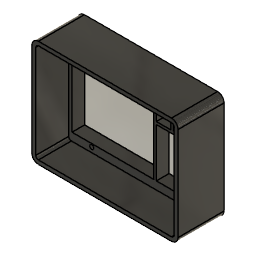
Fibonnaci Body (Autodesk Fusion 360 design; units mm, degrees)
Autodesk Fusion 360 part; units mm, degrees
sketch "Sketch1" plane through (0, 0, 0) normal (0, 1, 0) x (1, 0, 0)
  line L0 (-88.7415, 32.8321) -> (-88.7415, 21.8321)
  line L1 (-88.7415, 21.8321) -> (-77.7415, 21.8321)
  line L2 (-77.7415, 21.8321) -> (-77.7415, 32.8321)
  line L3 (-77.7415, 32.8321) -> (-88.7415, 32.8321)
  line L4 (-77.7415, -30.168) -> (-77.7415, 6.8321)
  line L5 (-77.7415, 19.8321) -> (-88.7415, 19.8321)
  line L6 (-77.7415, 8.8321) -> (-77.7415, 19.8321)
  line L7 (-88.7415, 8.8321) -> (-77.7415, 8.8321)
  line L8 (-88.7415, 19.8321) -> (-88.7415, 8.8321)
  line L9 (-75.7414, 32.8321) -> (-75.7414, -30.168)
  line L10 (-90.7415, 8.8321) -> (-90.7415, 32.8321)
  line L11 (-75.7414, -30.168) -> (-13.7413, -30.168)
  line L12 (-113.7415, 8.8321) -> (-90.7415, 8.8321)
  line L13 (-77.7415, 6.8321) -> (-113.7415, 6.8321)
  line L14 (-90.7415, 32.8321) -> (-113.7415, 32.8321)
  line L15 (-113.7415, -30.168) -> (-77.7415, -30.168)
  line L16 (-13.7413, 32.8321) -> (-75.7414, 32.8321)
  line L17 (-13.7413, 32.8321) -> (-13.7413, -30.168)
  line L18 (-113.7415, 8.8321) -> (-113.7415, 32.8321)
  line L19 (-113.7415, -30.168) -> (-113.7415, 6.8321)
  arc A0 (-27.1914, -32.427) -> (-30.2914, -32.427) centre (-28.7414, -32.427) ccw
  arc A1 (-30.2914, -32.427) -> (-27.1914, -32.427) centre (-28.7414, -32.427) ccw
  arc A2 (-97.1915, -32.427) -> (-100.2915, -32.427) centre (-98.7415, -32.427) ccw
  arc A3 (-100.2915, -32.427) -> (-97.1915, -32.427) centre (-98.7415, -32.427) ccw
  arc A4 (-97.1915, 35.0863) -> (-100.2915, 35.0863) centre (-98.7415, 35.0863) ccw
  arc A5 (-100.2915, 35.0863) -> (-97.1915, 35.0863) centre (-98.7415, 35.0863) ccw
  arc A6 (-30.2914, 35.0863) -> (-27.1914, 35.0863) centre (-28.7414, 35.0863) ccw
  arc A7 (-27.1914, 35.0863) -> (-30.2914, 35.0863) centre (-28.7414, 35.0863) ccw
  line L20 (-118.7415, 6.8321) -> (-118.7415, 8.8321)
  line L21 (-12.7414, 33.8297) -> (-114.7414, 33.8297)
  line L22 (-114.7414, 33.8297) -> (-114.7414, -31.1703)
  line L23 (-114.7414, -31.1703) -> (-12.7414, -31.1703)
  line L24 (-12.7414, -31.1703) -> (-12.7414, 33.8297)
  line L25 (-114.2414, -39.1703) -> (-13.2414, -39.1703)
  line L26 (-8.2414, -34.1703) -> (-8.2414, 36.8297)
  line L27 (-13.2414, 41.8297) -> (-114.2414, 41.8297)
  line L28 (-119.2414, 36.8297) -> (-119.2414, -34.1703)
  arc A8 (-114.2414, 41.8297) -> (-119.2414, 36.8297) centre (-114.2414, 36.8297) ccw
  arc A9 (-8.2414, 36.8297) -> (-13.2414, 41.8297) centre (-13.2414, 36.8297) ccw
  arc A10 (-119.2414, -34.1703) -> (-114.2414, -39.1703) centre (-114.2414, -34.1703) ccw
  arc A11 (-13.2414, -39.1703) -> (-8.2414, -34.1703) centre (-13.2414, -34.1703) ccw
  point P0 (-63.7414, 1.3297)
  dimension "d10" = 102
  dimension "d11" = 65
  dimension "d15" = 5
  constraint horizontal L21
  constraint perpendicular L21 L22
  constraint parallel L21 L23
  constraint parallel L22 L24
  constraint tangent L28 A8
  constraint tangent L27 A8
  constraint tangent L27 A9
  constraint tangent L26 A9
  constraint equal A8 A9
  constraint tangent L28 A10
  constraint tangent L25 A10
  constraint equal A8 A10
  constraint tangent L26 A11
  constraint tangent L25 A11
  constraint equal A8 A11
  measures "d10" distance of L22.end L23.end
  measures "d11" distance of L21.end L22.end
  measures "d15" radius of A8
extrude "Extrude4" add sketch "Sketch1" against normal blind 10 contours A0 A2 A5 A6 L21 L22 L23 L24 | L25 L26 L27 L28 A8 A9 A10 A11 makes body 1
extrude "Extrude5" add sketch "Sketch1" against normal blind 0.4 separate body contours L9 L11 L16 L17 makes body 2
extrude "Extrude6" add sketch "Sketch1" against normal blind 0.4 separate body contours L0 L1 L2 L3 makes body 3
extrude "Extrude7" add sketch "Sketch1" against normal blind 0.4 separate body contours L10 L12 L14 L18 makes body 4
extrude "Extrude8" add sketch "Sketch1" against normal blind 0.4 separate body contours L5 L6 L7 L8 makes body 5
extrude "Extrude9" add sketch "Sketch1" against normal blind 0.4 separate body contours L4 L13 L15 L19 makes body 6
extrude "Extrude10" add sketch "Sketch1" against normal blind 15 contours A0 A1 L23 | A0 L23 | A2 L23 | A2 A3 L23 | A6 A7 L21 | A6 L21 | A4 A5 L21 | A5 L21 bodies 1
sketch "Sketch6" plane through (0, -10, 0) normal (0, -1, 0) x (1, 0, 0)
  line L0 (-90.7415, -8.8321) -> (-90.7415, -32.8321)
  line L1 (-90.7415, -32.8321) -> (-113.7415, -32.8321)
  line L2 (-113.7415, -32.8321) -> (-113.7415, -8.8321)
  line L3 (-113.7415, -8.8321) -> (-90.7415, -8.8321)
  line L4 (-77.7415, 30.168) -> (-77.7415, -6.8321)
  line L5 (-77.7415, -6.8321) -> (-113.7415, -6.8321)
  line L6 (-113.7415, -6.8321) -> (-113.7415, 30.168)
  line L7 (-113.7415, 30.168) -> (-77.7415, 30.168)
  line L8 (-88.7415, -19.8321) -> (-88.7415, -8.8321)
  line L9 (-88.7415, -8.8321) -> (-77.7415, -8.8321)
  line L10 (-77.7415, -8.8321) -> (-77.7415, -19.8321)
  line L11 (-77.7415, -19.8321) -> (-88.7415, -19.8321)
  line L12 (-77.7415, -32.8321) -> (-88.7415, -32.8321)
  line L13 (-88.7415, -32.8321) -> (-88.7415, -21.8321)
  line L14 (-88.7415, -21.8321) -> (-77.7415, -21.8321)
  line L15 (-77.7415, -21.8321) -> (-77.7415, -32.8321)
  line L16 (-75.7414, -32.8321) -> (-75.7414, 30.168)
  line L17 (-75.7414, 30.168) -> (-13.7413, 30.168)
  line L18 (-13.7413, 30.168) -> (-13.7413, -32.8321)
  line L19 (-13.7413, -32.8321) -> (-75.7414, -32.8321)
  arc A0 (-8.2414, 34.1703) -> (-13.2414, 39.1703) centre (-13.2414, 34.1703) ccw
  line L20 (-13.2414, 39.1703) -> (-114.2414, 39.1703)
  arc A1 (-114.2414, 39.1703) -> (-119.2414, 34.1703) centre (-114.2414, 34.1703) ccw
  line L21 (-119.2414, 34.1703) -> (-119.2414, -36.8297)
  arc A2 (-119.2414, -36.8297) -> (-114.2414, -41.8297) centre (-114.2414, -36.8297) ccw
  line L22 (-114.2414, -41.8297) -> (-13.2414, -41.8297)
  arc A3 (-13.2414, -41.8297) -> (-8.2414, -36.8297) centre (-13.2414, -36.8297) ccw
  line L23 (-8.2414, -36.8297) -> (-8.2414, 34.1703)
  circle A4 centre (-28.7414, 32.427) radius 1.55
  circle A5 centre (-98.7415, 32.427) radius 1.55
  circle A6 centre (-28.7414, -35.0863) radius 1.55
  circle A7 centre (-98.7415, -35.0863) radius 1.55
sketch "Sketch7" plane through (0, -10, 0) normal (0, -1, 0) x (1, 0, 0)
  line L0 (-90.7415, -8.8321) -> (-90.7415, -32.8321)
  line L1 (-90.7415, -32.8321) -> (-113.7415, -32.8321)
  line L2 (-113.7415, -32.8321) -> (-113.7415, -8.8321)
  line L3 (-113.7415, -8.8321) -> (-90.7415, -8.8321)
  line L4 (-77.7415, 30.168) -> (-77.7415, -6.8321)
  line L5 (-77.7415, -6.8321) -> (-113.7415, -6.8321)
  line L6 (-113.7415, -6.8321) -> (-113.7415, 30.168)
  line L7 (-113.7415, 30.168) -> (-77.7415, 30.168)
  line L8 (-88.7415, -19.8321) -> (-88.7415, -8.8321)
  line L9 (-88.7415, -8.8321) -> (-77.7415, -8.8321)
  line L10 (-77.7415, -8.8321) -> (-77.7415, -19.8321)
  line L11 (-77.7415, -19.8321) -> (-88.7415, -19.8321)
  line L12 (-77.7415, -32.8321) -> (-88.7415, -32.8321)
  line L13 (-88.7415, -32.8321) -> (-88.7415, -21.8321)
  line L14 (-88.7415, -21.8321) -> (-77.7415, -21.8321)
  line L15 (-77.7415, -21.8321) -> (-77.7415, -32.8321)
  line L16 (-75.7414, -32.8321) -> (-75.7414, 30.168)
  line L17 (-75.7414, 30.168) -> (-13.7413, 30.168)
  line L18 (-13.7413, 30.168) -> (-13.7413, -32.8321)
  line L19 (-13.7413, -32.8321) -> (-75.7414, -32.8321)
  arc A0 (-8.2414, 34.1703) -> (-13.2414, 39.1703) centre (-13.2414, 34.1703) ccw
  line L20 (-13.2414, 39.1703) -> (-114.2414, 39.1703)
  arc A1 (-114.2414, 39.1703) -> (-119.2414, 34.1703) centre (-114.2414, 34.1703) ccw
  line L21 (-119.2414, 34.1703) -> (-119.2414, -36.8297)
  arc A2 (-119.2414, -36.8297) -> (-114.2414, -41.8297) centre (-114.2414, -36.8297) ccw
  line L22 (-114.2414, -41.8297) -> (-13.2414, -41.8297)
  arc A3 (-13.2414, -41.8297) -> (-8.2414, -36.8297) centre (-13.2414, -36.8297) ccw
  line L23 (-8.2414, -36.8297) -> (-8.2414, 34.1703)
  line L24 (-11.2414, -36.8297) -> (-11.2414, 34.1703)
  arc A4 (-11.2414, 34.1703) -> (-13.2414, 36.1703) centre (-13.2414, 34.1703) ccw
  line L25 (-13.2414, 36.1703) -> (-114.2414, 36.1703)
  arc A5 (-114.2414, 36.1703) -> (-116.2414, 34.1703) centre (-114.2414, 34.1703) ccw
  line L26 (-116.2414, 34.1703) -> (-116.2414, -36.8297)
  arc A6 (-116.2414, -36.8297) -> (-114.2414, -38.8297) centre (-114.2414, -36.8297) ccw
  line L27 (-114.2414, -38.8297) -> (-13.2414, -38.8297)
  arc A7 (-13.2414, -38.8297) -> (-11.2414, -36.8297) centre (-13.2414, -36.8297) ccw
  circle A8 centre (-28.7414, 32.427) radius 1.55
  circle A9 centre (-98.7415, 32.427) radius 1.55
  circle A10 centre (-28.7414, -35.0863) radius 1.55
  circle A11 centre (-98.7415, -35.0863) radius 1.55
  dimension "d32" = -3
extrude "Extrude11" add sketch "Sketch7" along normal blind 25 contours A0 L20 A1 L21 A2 L22 A3 L23 bodies 1
sketch "Sketch8" plane through (0, -35, 0) normal (0, -1, 0) x (1, 0, 0)
  arc A0 (-13.2414, -38.8297) -> (-11.2414, -36.8297) centre (-13.2414, -36.8297) ccw
  line L0 (-13.2414, -38.8297) -> (-114.2414, -38.8297)
  arc A1 (-116.2414, -36.8297) -> (-114.2414, -38.8297) centre (-114.2414, -36.8297) ccw
  line L1 (-116.2414, -36.8297) -> (-116.2414, 34.1703)
  arc A2 (-114.2414, 36.1703) -> (-116.2414, 34.1703) centre (-114.2414, 34.1703) ccw
  line L2 (-114.2414, 36.1703) -> (-13.2414, 36.1703)
  arc A3 (-11.2414, 34.1703) -> (-13.2414, 36.1703) centre (-13.2414, 34.1703) ccw
  line L3 (-11.2414, 34.1703) -> (-11.2414, -36.8297)
  line L4 (-8.2414, -36.8297) -> (-8.2414, 34.1703)
  arc A4 (-8.2414, 34.1703) -> (-13.2414, 39.1703) centre (-13.2414, 34.1703) ccw
  line L5 (-13.2414, 39.1703) -> (-114.2414, 39.1703)
  arc A5 (-114.2414, 39.1703) -> (-119.2414, 34.1703) centre (-114.2414, 34.1703) ccw
  line L6 (-119.2414, 34.1703) -> (-119.2414, -36.8297)
  arc A6 (-119.2414, -36.8297) -> (-114.2414, -41.8297) centre (-114.2414, -36.8297) ccw
  line L7 (-114.2414, -41.8297) -> (-13.2414, -41.8297)
  arc A7 (-13.2414, -41.8297) -> (-8.2414, -36.8297) centre (-13.2414, -36.8297) ccw
sketch "Sketch9" plane through (0, -35, 0) normal (0, -1, 0) x (1, 0, 0)
  arc A0 (-13.2414, -38.8297) -> (-11.2414, -36.8297) centre (-13.2414, -36.8297) ccw
  line L0 (-13.2414, -38.8297) -> (-114.2414, -38.8297)
  arc A1 (-116.2414, -36.8297) -> (-114.2414, -38.8297) centre (-114.2414, -36.8297) ccw
  line L1 (-116.2414, -36.8297) -> (-116.2414, 34.1703)
  arc A2 (-114.2414, 36.1703) -> (-116.2414, 34.1703) centre (-114.2414, 34.1703) ccw
  line L2 (-114.2414, 36.1703) -> (-13.2414, 36.1703)
  arc A3 (-11.2414, 34.1703) -> (-13.2414, 36.1703) centre (-13.2414, 34.1703) ccw
  line L3 (-11.2414, 34.1703) -> (-11.2414, -36.8297)
  line L4 (-8.2414, -36.8297) -> (-8.2414, 34.1703)
  arc A4 (-8.2414, 34.1703) -> (-13.2414, 39.1703) centre (-13.2414, 34.1703) ccw
  line L5 (-13.2414, 39.1703) -> (-114.2414, 39.1703)
  arc A5 (-114.2414, 39.1703) -> (-119.2414, 34.1703) centre (-114.2414, 34.1703) ccw
  line L6 (-119.2414, 34.1703) -> (-119.2414, -36.8297)
  arc A6 (-119.2414, -36.8297) -> (-114.2414, -41.8297) centre (-114.2414, -36.8297) ccw
  line L7 (-114.2414, -41.8297) -> (-13.2414, -41.8297)
  arc A7 (-13.2414, -41.8297) -> (-8.2414, -36.8297) centre (-13.2414, -36.8297) ccw
  line L8 (-11.2414, -36.8297) -> (-11.2414, 34.1703)
  arc A8 (-11.2414, 34.1703) -> (-13.2414, 36.1703) centre (-13.2414, 34.1703) ccw
  line L9 (-13.2414, 36.1703) -> (-114.2414, 36.1703)
  arc A9 (-114.2414, 36.1703) -> (-116.2414, 34.1703) centre (-114.2414, 34.1703) ccw
  line L10 (-116.2414, 34.1703) -> (-116.2414, -36.8297)
  arc A10 (-116.2414, -36.8297) -> (-114.2414, -38.8297) centre (-114.2414, -36.8297) ccw
  line L11 (-114.2414, -38.8297) -> (-13.2414, -38.8297)
  arc A11 (-13.2414, -38.8297) -> (-11.2414, -36.8297) centre (-13.2414, -36.8297) ccw
  line L12 (-90.7415, -8.8321) -> (-90.7415, -32.8321)
  line L13 (-90.7415, -32.8321) -> (-113.7415, -32.8321)
  line L14 (-113.7415, -32.8321) -> (-113.7415, -8.8321)
  line L15 (-113.7415, -8.8321) -> (-90.7415, -8.8321)
  line L16 (-77.7415, 30.168) -> (-77.7415, -6.8321)
  line L17 (-77.7415, -6.8321) -> (-113.7415, -6.8321)
  line L18 (-113.7415, -6.8321) -> (-113.7415, 30.168)
  line L19 (-113.7415, 30.168) -> (-77.7415, 30.168)
  line L20 (-88.7415, -19.8321) -> (-88.7415, -8.8321)
  line L21 (-88.7415, -8.8321) -> (-77.7415, -8.8321)
  line L22 (-77.7415, -8.8321) -> (-77.7415, -19.8321)
  line L23 (-77.7415, -19.8321) -> (-88.7415, -19.8321)
  line L24 (-77.7415, -32.8321) -> (-88.7415, -32.8321)
  line L25 (-88.7415, -32.8321) -> (-88.7415, -21.8321)
  line L26 (-88.7415, -21.8321) -> (-77.7415, -21.8321)
  line L27 (-77.7415, -21.8321) -> (-77.7415, -32.8321)
  line L28 (-75.7414, -32.8321) -> (-75.7414, 30.168)
  line L29 (-75.7414, 30.168) -> (-13.7413, 30.168)
  line L30 (-13.7413, 30.168) -> (-13.7413, -32.8321)
  line L31 (-13.7413, -32.8321) -> (-75.7414, -32.8321)
  circle A12 centre (-28.7414, 32.427) radius 1.55
  circle A13 centre (-98.7415, 32.427) radius 1.55
  circle A14 centre (-28.7414, -35.0863) radius 1.55
  circle A15 centre (-98.7415, -35.0863) radius 1.55
sketch "Sketch10" plane through (0, 0, 36.1703) normal (0, 0, -1) x (1, 0, 0)
  line L0 (-114.2414, 10) -> (-13.2414, 10)
  line L1 (-13.2414, 10) -> (-13.2414, 35)
  line L2 (-13.2414, 35) -> (-114.2414, 35)
  line L3 (-114.2414, 35) -> (-114.2414, 10)
sketch "Sketch11" plane through (0, 0, 0) normal (0, 1, 0) x (-1, 0, 0)
  line L0 (90.7415, -8.8321) -> (90.7415, -32.8321)
  line L1 (90.7415, -32.8321) -> (113.7415, -32.8321)
  line L2 (113.7415, -32.8321) -> (113.7415, -8.8321)
  line L3 (113.7415, -8.8321) -> (90.7415, -8.8321)
  line L4 (86.0498, -3.57) -> (43.2213, -4.4417) construction
  line L5 (43.2213, -4.4417) -> (43.7849, -32.1345) construction
  line L6 (43.7849, -32.1345) -> (86.6134, -31.2628) construction
  line L7 (86.6134, -31.2628) -> (86.0498, -3.57) construction
  dimension "d39" = 8
  dimension "d40" = 0
sketch "Sketch12" plane through (0, 0, 36.1703) normal (0, 0, -1) x (1, 0, 0)
  line L0 (-114.2414, 10) -> (-13.2414, 10)
  line L1 (-13.2414, 10) -> (-13.2414, 35)
  line L2 (-13.2414, 35) -> (-114.2414, 35)
  line L3 (-114.2414, 35) -> (-114.2414, 10)
extrude "Extrude12" cut 4 faces at (-28.6264, -15, -34.5826) (-98.7801, -15, -35.6016) (-28.2656, -15, 32.0115) (-98.7801, -15, 31.9118) along direction (0, 1, 0) blind 10 on bodies 1 bodies 1
sketch "Sketch13" plane through (0, 0, 36.1703) normal (0, 0, -1) x (1, 0, 0)
  line L0 (-114.2414, 10) -> (-13.2414, 10)
  line L1 (-13.2414, 10) -> (-13.2414, 35)
  line L2 (-13.2414, 35) -> (-114.2414, 35)
  line L3 (-114.2414, 35) -> (-114.2414, 10)
sketch "Sketch14" plane through (0, 0, -32.8321) normal (0, 0, 1) x (-1, 0, 0)
  line L0 (13.7413, 0) -> (75.7414, 0)
  line L1 (75.7414, 0) -> (75.7414, 10)
  line L2 (75.7414, 10) -> (13.7413, 10)
  line L3 (13.7413, 10) -> (13.7413, 0)
sketch "Sketch15" plane through (0, 0, 39.1703) normal (0, 0, 1) x (-1, 0, 0)
  line L0 (13.2414, 0) -> (114.2414, 0)
  line L1 (114.2414, 0) -> (114.2414, 35)
  line L2 (114.2414, 35) -> (13.2414, 35)
  line L3 (13.2414, 35) -> (13.2414, 0)
move_body "Move1" bodies 1 2 3 4 6 5 to x (-1, 0, 0) y (0, 1, 0) z (0, 0, -1) at (-238.4828, 0, -83.6593)
move_body "Move2" bodies 1 2 3 4 6 5 to x (1, 0, 0) y (0, 1, 0) z (0, 0, 1) at (125, -50, 75)
equation "d40 = '1'"
